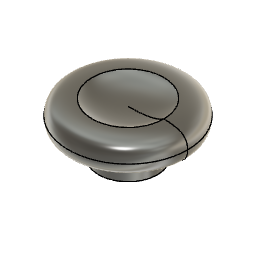
Joystickaufsatz v4 (Autodesk Fusion 360 design; units mm, degrees)
Autodesk Fusion 360 part; units mm, degrees
sketch "Skizze1" plane through (0, 0, 0) normal (0, 1, 0) x (1, 0, 0)
  line L0 (0, 0) -> (3.1, 0)
  line L1 (3.1, 0) -> (3.1, -10)
  line L2 (3.1, -10) -> (0, -10)
  line L3 (0, -10) -> (0, 0)
  line L4 (0, 0) -> (4.1, 0)
  line L5 (4.1, 0) -> (4.1, -11)
  line L6 (4.1, -11) -> (0, -11)
  line L7 (0, -11) -> (0, 0)
  spline S0 degree 5 poles (4.1, -11) (4.2279, -10.9985) (4.4788, -10.9973) (4.8407, -11.0005) (5.2943, -11.0151) (5.8115, -11.0509) (6.2773, -11.1052) (6.6899, -11.1789) (7.0481, -11.2731) (7.3523, -11.3889) (7.6051, -11.5265) (7.8109, -11.6864) (7.9746, -11.8685) (8.1014, -12.0725) (8.1954, -12.2979) (8.2598, -12.5439) (8.2891, -12.7567) (8.2992, -12.925) (8.3006, -13.041) (8.3, -13.1) knots 0 0 0 0 0 0 0.066667 0.133333 0.2 0.266667 0.333333 0.4 0.466667 0.533333 0.6 0.666667 0.733333 0.8 0.866667 0.933333 1 1 1 1 1 1
  spline S1 degree 5 poles (4.1, -15.2) (4.2279, -15.2015) (4.4788, -15.2027) (4.8407, -15.1995) (5.2943, -15.1849) (5.8115, -15.1491) (6.2773, -15.0948) (6.6899, -15.0211) (7.0481, -14.9269) (7.3523, -14.8111) (7.6051, -14.6735) (7.8109, -14.5136) (7.9746, -14.3315) (8.1014, -14.1275) (8.1954, -13.9021) (8.2598, -13.6561) (8.2891, -13.4433) (8.2992, -13.275) (8.3006, -13.159) (8.3, -13.1) knots 0 0 0 0 0 0 0.066667 0.133333 0.2 0.266667 0.333333 0.4 0.466667 0.533333 0.6 0.666667 0.733333 0.8 0.866667 0.933333 1 1 1 1 1 1
  line L8 (3.3404, -11.0087) -> (4.8596, -10.9913)
  line L9 (8.3067, -12.4468) -> (8.2933, -13.7532)
  line L10 (3.3404, -15.1913) -> (4.8596, -15.2087)
  line L11 (8.3067, -13.7532) -> (8.2933, -12.4468)
  line L12 (4.1, -15.2) -> (0, -15.2)
  line L13 (0, -15.2) -> (0, -11)
  spline S2 degree 5 poles (4.9999, -15.192) (4.9392, -15.1524) (4.8142, -15.0748) (4.616, -14.964) (4.3298, -14.8273) (3.9334, -14.6758) (3.4953, -14.5454) (3.013, -14.4373) (2.4867, -14.3514) (1.9196, -14.286) (1.3152, -14.2394) (0.8048, -14.2158) (0.4078, -14.2052) (0.137, -14.2012) (0, -14.2) knots 0 0 0 0 0 0 0.1 0.2 0.3 0.4 0.5 0.6 0.7 0.8 0.9 1 1 1 1 1 1
  point P0 (7.1, -11.3)
  point P1 (8.05, -12)
  point P2 (7.1, -14.9)
  point P3 (8.05, -14.2)
  point P4 (3.2286, -14.4897)
  dimension "d1" = 3.1
  dimension "d2" = 10
  dimension "d3" = 4.1
  dimension "d4" = 11
  constraint horizontal L0
  constraint vertical L1
  constraint horizontal L2
  constraint vertical L3
  constraint coincident L0.start L3.end
  constraint horizontal L4
  constraint vertical L5
  constraint horizontal L6
  constraint vertical L7
  constraint midpoint L5.end L8
  constraint midpoint S0.end L9
  constraint horizontal L12
  constraint perpendicular L6 L13
  constraint coincident S1 S2.start
  constraint coincident L13 S2.end
  measures "d1" distance of L0.start L0.end
  measures "d2" distance of L0.start L2.end
  measures "d3" distance of L0.start L4.end
  measures "d4" distance of L0.start L6.end
revolve "Drehen1" add sketch "Skizze1" angle 360 about axis through (0, 0, 10) along (0, 0, -1) contours L1 L2 L4 L5 L6 L7 | L6 S0 S1 L13 S2
extrude "Extrusion1" cut 1 faces at (0.3965, -0.7189, 10) along direction (0, 0, 1) blind 3
extrude "Extrusion2" cut 1 faces at (3.7514, 0.2037, 0) along direction (0, 0, 1) blind 3
move_body "Verschieben1" bodies 1 to x (1, 0, 0) y (0, 1, 0) z (0, 0, 1) at (0, 0, -3)
extrude "Extrusion3" cut 1 faces at (3.7514, 0.2037, 0) along direction (0, 0, 1) blind 5
move_body "Verschieben2" bodies 1 to x (1, 0, 0) y (0, 1, 0) z (0, 0, 1) at (-0.0556, -0.1501, -4.9974)
move_body "Verschieben3" bodies 1 to x (1, 0, 0) y (0, 1, 0) z (0, 0, 1) at (0.0556, 0.1501, -5.0026)
move_body "Verschieben4" bodies 1 to x (1, 0, 0) y (0, 1, 0) z (0, 0, 1) at (0, 0, 5)
sketch "Skizze2" plane through (0, 0, 5) normal (0, 0, -1) x (1, 0, 0)
  circle A0 centre (0, 0) radius 3.1
  circle A1 centre (0, 0) radius 3.05
  dimension "d12" = 6.1
  constraint coincident A0.centre A1.centre
  measures "d12" diameter of A1
extrude "Extrusion4" add sketch "Skizze2" along normal up to surface (5 mm away)
